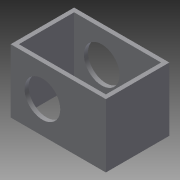
# Autodesk Inventor part: Hinge
Saved by Autodesk Inventor 2015 (Build 190159000, 159)
## iProperties
Created: 2015-01-29
Part Number: Hinge
Material: Generic
Document SubType Name: Modeling
Designer: pltwe4
Density: 1 g/cm^3
Appearance: Default
Author: pltwe4
Autodesk Inventor part; units mm, degrees
ref_plane "YZ Plane" through (0, 0, 0) normal (1, 0, 0) x (0, 1, 0)
ref_plane "XZ Plane" through (0, 0, 0) normal (0, 1, 0) x (-1, 0, 0)
ref_plane "XY Plane" through (0, 0, 0) normal (0, 0, 1) x (1, 0, 0)
sketch "Sketch1" plane through (0, 0, 0) normal (0, 1, 0) x (-1, 0, 0)
  point P0 (0, 0)
sketch "Sketch2" plane through (0, 0, 0) normal (0, 1, 0) x (-1, 0, 0)
  line L0 (38.1, 25.4) -> (-38.1, 25.4)
  line L1 (-38.1, 25.4) -> (-38.1, -25.4)
  line L2 (-38.1, -25.4) -> (38.1, -25.4)
  line L3 (38.1, -25.4) -> (38.1, 25.4)
  line L4 (34.798, 22.098) -> (-34.798, 22.098)
  line L5 (-34.798, 22.098) -> (-34.798, -22.098)
  line L6 (-34.798, -22.098) -> (34.798, -22.098)
  line L7 (34.798, -22.098) -> (34.798, 22.098)
  line L8 (0, -35.56) -> (0, 35.56) projected
  line L9 (-53.34, 0) -> (53.34, 0) projected
  point P0 (0, 0)
  dimension "d0" = 3.302
  dimension "d1" = 76.2
  dimension "d2" = 50.8
  constraints: 16 end point, 4 parallel, 2 perpendicular, 1 horizontal, 5 other
  measures "d0" distance between parallel lines of L7 L3
  measures "d1" distance between parallel lines of L1 L3
  measures "d2" distance between parallel lines of L0 L2
extrude "Extrusion1" add sketch "Sketch2" along normal mid plane 50.8 contours L3 L9 L7 L4 L8 L0 | L8 L4 L5 L9 L1 L0 | L3 L2 L8 L6 L7 L9 | L9 L5 L6 L8 L2 L1
sketch "Sketch3" plane through (-38.1, -25.4, 25.4) normal (0, 0, 1) x (1, 0, 0)
  circle A0 centre (25.4, 25.4) radius 14.2875
  line L0 (-15.24, 25.4) -> (91.44, 25.4) projected
  line L1 (38.1, 60.96) -> (38.1, -10.16) projected
  line L2 (0, 50.8) -> (0, 0) projected
  point P0 (38.1, 25.4)
  dimension "d5" = 28.575
  dimension "d6" = 25.4
  constraints: 1 centre point, 1 point on line
  measures "d5" diameter of A0
  measures "d6" distance from line of L2 A0.centre
extrude "Extrusion2" cut sketch "Sketch3" against normal up to surface (50.8 mm away)
body "Solid1"
